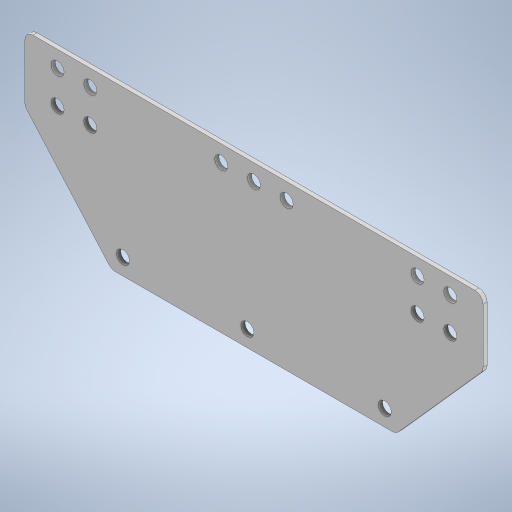
# Autodesk Inventor part: wedge
Saved by Autodesk Inventor 2023 (Build 270158000, 158)
## iProperties
Created: 2023-12-11
Part Number: wedge
Material: Generic
Document SubType Name: Modeling
Designer: Meer
Density: 1 g/cm^3
Appearance: Default
Author: Meer
Autodesk Inventor part; units mm, degrees
ref_plane "YZ Plane" through (0, 0, 0) normal (1, 0, 0) x (0, 1, 0)
ref_plane "XZ Plane" through (0, 0, 0) normal (0, 1, 0) x (-1, 0, 0)
ref_plane "XY Plane" through (0, 0, 0) normal (0, 0, 1) x (1, 0, 0)
sketch "Sketch1" plane through (0, 0, 0) normal (0, 0, 1) x (1, 0, 0)
  line L0 (-83.8471, 83.8315) -> (93.9529, 83.8315)
  line L1 (93.9529, 83.8315) -> (93.9529, 20.3315)
  line L2 (93.9529, 20.3315) -> (-83.8471, 20.3315)
  line L3 (-83.8471, 20.3315) -> (-83.8471, 83.8315)
  line L4 (-83.8471, 20.3315) -> (-83.8471, 58.4315)
  line L5 (93.9529, 20.3315) -> (93.9529, 58.2798)
  line L6 (93.9529, 58.2798) -> (60.1807, 20.3315)
  line L7 (-83.8471, 58.4315) -> (-50.246, 20.3315)
  circle A0 centre (-58.4471, 77.4815) radius 2.54
  circle A1 centre (68.5529, 77.4815) radius 2.54
  circle A2 centre (2.5129, 26.6815) radius 2.54
  circle A3 centre (-45.7471, 26.6815) radius 2.54
  circle A4 centre (55.8529, 26.6815) radius 2.54
  line L8 (-58.4471, 77.4815) -> (-71.1471, 77.4815)
  circle A5 centre (-71.1471, 77.4815) radius 2.54
  line L9 (-71.1471, 77.4815) -> (-71.1471, 64.7815)
  line L10 (-71.1471, 64.7815) -> (-58.4471, 64.7815)
  circle A6 centre (-71.1471, 64.7815) radius 2.54
  circle A7 centre (-58.4471, 64.7815) radius 2.54
  line L11 (-58.4471, 77.4815) -> (5.0529, 77.4815)
  line L12 (5.0529, 77.4815) -> (-7.6471, 77.4815)
  circle A8 centre (-7.6471, 77.4815) radius 2.54
  circle A9 centre (5.0529, 77.4815) radius 2.54
  line L13 (5.0529, 77.4815) -> (17.7529, 77.4815)
  circle A10 centre (17.7529, 77.4815) radius 2.54
  line L14 (68.5529, 77.4815) -> (81.2529, 77.4815)
  line L15 (81.2529, 77.4815) -> (81.2529, 64.7815)
  line L16 (81.2529, 64.7815) -> (68.5529, 64.7815)
  circle A11 centre (81.2529, 77.4815) radius 2.54
  circle A12 centre (81.2529, 64.7815) radius 2.54
  circle A13 centre (68.5529, 64.7815) radius 2.54
  point P0 (0, 0)
  dimension "d0" = 177.8
  dimension "d1" = 63.5
  dimension "d2" = 38.1
  dimension "d3" = 50.8
  dimension "d4" = 50.8
  dimension "d18" = 6.35
  dimension "d19" = 25.4
  dimension "d20" = 5.08
  dimension "d21" = 5.08
  dimension "d22" = 6.35
  dimension "d23" = 25.4
  dimension "d24" = 5.08
  dimension "d25" = 6.35
  dimension "d26" = 86.36
  dimension "d29" = 6.35
  dimension "d30" = 6.35
  dimension "d31" = 38.1
  dimension "d32" = 38.1
  dimension "d33" = 5.08
  dimension "d34" = 5.08
  dimension "d39" = 12.7
  dimension "d40" = 5.08
  dimension "d41" = 12.7
  dimension "d42" = 5.08
  dimension "d43" = 5.08
  dimension "d44" = 12.7
  dimension "d45" = 5.08
  dimension "d46" = 5.08
  dimension "d47" = 12.7
  dimension "d48" = 5.08
  dimension "d49" = 12.7
  dimension "d50" = 12.7
  dimension "d51" = 12.7
  dimension "d52" = 5.08
  dimension "d53" = 5.08
  dimension "d54" = 5.08
  constraints: 34 end point, 14 centre point, 9 coincident, 5 horizontal, 5 point on line, 4 perpendicular, 2 parallel, 1 vertical
  measures "d0" distance of L0.start L0.end
  measures "d1" distance of L0.end L1.end
  measures "d2" distance of L2.end L4.end
  measures "d3" distance of L5.end L6.end
  measures "d4" distance of L4.end L7.end
  measures "d18" distance from line of L0 L8.start
  measures "d19" distance from line of L3 L8.start
  measures "d20" diameter of A0
  measures "d21" diameter of A1
  measures "d22" distance from line of L0 L14.start
  measures "d23" distance from line of L1 L14.start
  measures "d24" diameter of A2
  measures "d25" distance from line of L2 A2.centre
  measures "d26" distance from line of L3 A2.centre
  measures "d29" distance from line of L2 A4.centre
  measures "d30" distance from line of L2 A3.centre
  measures "d31" distance from line of L3 A3.centre
  measures "d32" distance from line of L1 A4.centre
  measures "d33" diameter of A3
  measures "d34" diameter of A4
  measures "d39" distance of L8.start L8.end
  measures "d40" diameter of A5
  measures "d41" distance of L9.start L9.end
  measures "d42" diameter of A6
  measures "d43" diameter of A7
  measures "d44" distance of L11.end L12.end
  measures "d45" diameter of A8
  measures "d46" diameter of A9
  measures "d47" distance of L13.start L13.end
  measures "d48" diameter of A10
  measures "d49" distance of L14.start L14.end
  measures "d50" distance of L14.end L15.end
  measures "d51" distance of L15.end L16.end
  measures "d52" diameter of A11
  measures "d53" diameter of A12
  measures "d54" diameter of A13
extrude "Extrusion3" add sketch "Sketch1" along normal blind 1.5875 contours L0 L1 L6 L2 L7 L3
fillet "Fillet6" radius 3.175 4 edges at (-83.8471, 58.4315, 0.7937) (-50.246, 20.3315, 0.7937) (60.1807, 20.3315, 0.7937) (-83.8471, 83.8315, 0.7937)
fillet "Fillet7" radius 3.175 2 edges at (93.9529, 83.8315, 0.7937) (93.9529, 58.2798, 0.7937)
body "Solid3"
